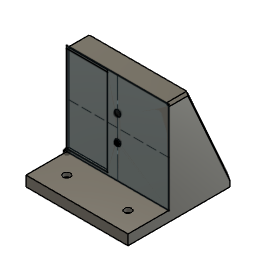
CNC_cable_guide_chain_holder (Autodesk Fusion 360 design; units mm, degrees)
Autodesk Fusion 360 part; units mm, degrees
note: some values were not read from the file. Set by a fixed rule: which sketch regions a step uses.
sketch "Sketch1" plane through (0, 0, 0) normal (0, 1, 0) x (1, 0, 0)
  line L0 (30, 30) -> (-30, 30)
  line L1 (-30, 30) -> (-30, -30)
  line L2 (-30, -30) -> (30, -30)
  line L3 (30, -30) -> (30, 30)
  line L4 (30, 30) -> (-30, -30) construction
  line L5 (-30, 30) -> (30, -30) construction
  circle A0 centre (-30, 30) radius 2.5
  circle A1 centre (30, 30) radius 2.5
  circle A2 centre (-30, -30) radius 2.5
  circle A3 centre (30, -30) radius 2.5
  line L6 (50, 50) -> (-50, 50)
  line L7 (-50, 50) -> (-50, -50)
  line L8 (-50, -50) -> (50, -50)
  line L9 (50, -50) -> (50, 50)
  line L10 (50, 50) -> (-50, -50) construction
  line L11 (-50, 50) -> (50, -50) construction
  line L12 (50, 10) -> (-50, 10)
  line L13 (-50, 10) -> (-50, -10)
  line L14 (-50, -10) -> (50, -10)
  line L15 (50, -10) -> (50, 10)
  line L16 (50, 10) -> (-50, -10) construction
  line L17 (-50, 10) -> (50, -10) construction
  circle A4 centre (-30, -30) radius 3.5
  circle A5 centre (30, -30) radius 3.5
  dimension "d1" = 60
  dimension "d2" = 60
  dimension "d3" = 5
  dimension "d6" = 60
  dimension "d7" = -60
  dimension "d8" = 100
  dimension "d9" = 100
  dimension "d10" = 100
  dimension "d11" = 20
  dimension "d49" = 7
  dimension "d50" = 7
  constraint horizontal L0
  constraint perpendicular L0 L1
  constraint parallel L0 L2
  constraint parallel L1 L3
  constraint coincident L4 origin
  constraint coincident L5 origin
  constraint coincident L0.end L1.start
  constraint horizontal L6
  constraint perpendicular L6 L7
  constraint parallel L6 L8
  constraint parallel L7 L9
  constraint coincident L10 origin
  constraint coincident L11 origin
  constraint horizontal L12
  constraint perpendicular L12 L13
  constraint parallel L12 L14
  constraint parallel L13 L15
  constraint coincident L16 origin
  constraint coincident L17 origin
  constraint coincident L1.end L2.start
  constraint concentric A3 A5
  measures "d1" distance of L1.end L2.end
  measures "d2" distance of L0.end L1.end
  measures "d3" diameter of A0
  measures "d8" distance of L7.end L8.end
  measures "d9" distance of L6.end L7.end
  measures "d10" distance of L13.end L14.end
  measures "d11" distance of L12.end L13.end
  measures "d49" diameter of A4
  measures "d50" diameter of A5
extrude "Extrude1" add sketch "Sketch1" along normal blind 10 contours L0 L1 L3 A0 A1 L6 L7 L9 L12 | L0 L1 L3 A0 A1 L12 | L1 L3 L12 L14 | L1 L7 L12 L13 L14 | L3 L9 L12 L14 L15 | L1 L2 L3 L14 A4 A5 | L1 L2 L3 L7 L8 L9 L14 A4 A5 | L1 L2 A2 A4 | L1 L2 A2 A4 | L2 L3 A3 A5 | L2 L3 A3 A5
extrude "Extrude2" add sketch "Sketch1" along normal blind 90 from surface at 10 contours L1 L3 L12 L14 | L1 L7 L12 L13 L14 | L3 L9 L12 L14 L15
sketch "Sketch2" plane through (0, 0, -10) normal (0, 0, -1) x (-1, 0, 0)
  line L0 (-50, 10) -> (50, 10)
  line L1 (50, 10) -> (50, 100)
  line L2 (50, 100) -> (-50, 100)
  line L3 (-50, 100) -> (-50, 10)
  line L4 (-50, 100) -> (-40, 100)
  line L5 (-40, 100) -> (-40, 10)
  line L6 (-40, 10) -> (-50, 10)
  line L7 (-50, 10) -> (-50, 100)
  line L8 (50, 100) -> (40, 100)
  line L9 (40, 100) -> (40, 10)
  line L10 (40, 10) -> (50, 10)
  line L11 (50, 10) -> (50, 100)
  line L12 (0, 100) -> (0, 10)
  line L13 (10, 100) -> (-10, 100)
  line L14 (-10, 100) -> (-10, 10)
  line L15 (-10, 10) -> (10, 10)
  line L16 (10, 10) -> (10, 100)
  dimension "d17" = 10
  dimension "d19" = 10
  dimension "d22" = 20
  dimension "d23" = 20
  constraint horizontal L4
  constraint vertical L5
  constraint horizontal L6
  constraint vertical L7
  constraint coincident L2.end L3.start
  constraint horizontal L8
  constraint vertical L9
  constraint horizontal L10
  constraint vertical L11
  constraint coincident L1.end L2.start
  constraint midpoint L2 L12.start
  constraint midpoint L0 L12.end
  constraint horizontal L13
  constraint vertical L14
  constraint horizontal L15
  constraint vertical L16
  constraint coincident L2 L13.start
  constraint collinear L0 L10
  constraint collinear L0 L15
  constraint collinear L0 L6
  measures "d17" distance of L2.end L4.end
  measures "d19" distance of L1.end L8.end
  measures "d23" distance of L13.start L13.end
extrude "Extrude3" add sketch "Sketch2" along normal up to surface (40 mm away) contours L0 L2 L3 L4 L5 L6 L7 | L0 L2 L12 L13 L14 L15 | L0 L2 L12 L13 L15 L16 | L0 L1 L2 L8 L9 L10 L11
chamfer "Chamfer1" distance 40 distance2 90 3 edges at (45, 100, -50) (0, 100, -50) (-45, 100, -50) measured on face at (-3.3333, 100, 3.3333) measured on face at (-3.3333, 100, 3.3333) measured on face at (-3.3333, 100, 3.3333)
chamfer "Chamfer2" distance 2.5 distance2 2 6 edges at (50, 55, -30) (40, 55, -30) (10, 55, -30) (-10, 55, -30) (-40, 55, -30) (-50, 55, -30) measured on face at (43.3333, 40, -36.6667) measured on face at (43.3333, 40, -36.6667) measured on face at (3.3333, 40, -36.6667) measured on face at (3.3333, 40, -36.6667) measured on face at (-43.3333, 70, -23.3333) measured on face at (-43.3333, 70, -23.3333)
chamfer "Chamfer3" distance 2.5 distance2 2 2 edges at (50, 100, 1.0943) (-50, 100, 1.0943) measured on face at (-2.5, 100, 3.3333) measured on face at (-50, 38.3585, -15.9371)
sketch "Sketch3" plane through (0, 0, 10) normal (0, 0, 1) x (1, 0, 0)
  line L0 (-48, 100) -> (-50, 97.5)
  line L1 (-50, 97.5) -> (-50, 10)
  line L2 (-50, 10) -> (50, 10)
  line L3 (50, 10) -> (50, 98)
  line L4 (50, 98) -> (47.5, 100)
  line L5 (47.5, 100) -> (-48, 100)
  line L6 (-0.25, 100) -> (0, 10)
  line L7 (-50, 10) -> (50, 10)
  line L8 (50, 10) -> (50, 100)
  line L9 (50, 100) -> (-50, 100)
  line L10 (-50, 100) -> (-50, 10)
  line L11 (50, 55) -> (-50, 55) construction
  circle A0 centre (-0.0903, 42.5) radius 2.8
  circle A1 centre (-0.0903, 67.5) radius 2.8
  line L12 (-50, 12.5) -> (-10.0903, 12.5)
  line L13 (-10.0903, 12.5) -> (-10.0903, 97.5)
  line L14 (-10.0903, 97.5) -> (-50, 97.5)
  line L15 (-50, 97.5) -> (-50, 12.5)
  dimension "d43" = 90
  dimension "d44" = 100
  dimension "d45" = 5.6
  dimension "d46" = 12.5
  dimension "d54" = 85
  dimension "d55" = 10
  constraint midpoint L5 L6.start
  constraint midpoint L2 L6.end
  constraint horizontal L7
  constraint vertical L8
  constraint horizontal L9
  constraint vertical L10
  constraint coincident L1.end L2.start
  constraint midpoint L8 L11.start
  constraint midpoint L10 L11.end
  constraint symmetric L11 A0 A1
  constraint coincident L6 A0.centre
  constraint horizontal L12
  constraint vertical L13
  constraint horizontal L14
  constraint vertical L15
  constraint symmetric L11 L12 L14
  constraint collinear L10 L15
  measures "d43" distance of L1.end L9.end
  measures "d44" distance of L8.end L9.end
  measures "d45" diameter of A0
  measures "d46" distance of L11 A0.centre
  measures "d54" distance of L12.start L0.end
  measures "d55" distance of A1.centre L13
extrude "Extrude4" cut sketch "Sketch3" against normal blind 8.1 contours L6 A1 | L6 A1 | L6 A0 | L6 A0
extrude "Extrude5" cut sketch "Sketch1" against normal blind 4 from surface at 10 contours L1 L2 A2 A4 | L1 L2 A2 A4 | L2 L3 A3 A5 | L2 L3 A3 A5
extrude "Extrude6" cut sketch "Sketch3" against normal blind 2 contours L1 L10 L12 L13 L14 L15
chamfer "Chamfer4" distance 2 angle 45 1 edges at (-30.0451, 97.5, 10)
equation "d46 = ( 25 / 2 ) * 1 mm"
